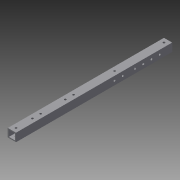
# Autodesk Inventor part: mounting block
Saved by Autodesk Inventor 2015 SP1 (Build 190203100, 203)
## iProperties
Created: 2015-01-16
Part Number: mounting block
Material: Generic
Document SubType Name: Modeling
Designer: Jarod
Density: 1 g/cm^3
Appearance: Default
Author: Jarod
Autodesk Inventor part; units mm, degrees
ref_plane "YZ Plane" through (0, 0, 0) normal (1, 0, 0) x (0, 1, 0)
ref_plane "XZ Plane" through (0, 0, 0) normal (0, 1, 0) x (-1, 0, 0)
ref_plane "XY Plane" through (0, 0, 0) normal (0, 0, 1) x (1, 0, 0)
sketch "Sketch1" plane through (0, 0, 0) normal (0, 0, 1) x (1, 0, 0)
  line L0 (0, 0) -> (25.4, 0)
  line L1 (25.4, 0) -> (25.4, 25.4)
  line L2 (25.4, 25.4) -> (0, 25.4)
  line L3 (0, 25.4) -> (0, 0)
  line L4 (3.175, 3.175) -> (22.225, 3.175)
  line L5 (22.225, 3.175) -> (22.225, 22.225)
  line L6 (22.225, 22.225) -> (3.175, 22.225)
  line L7 (3.175, 22.225) -> (3.175, 3.175)
  dimension "d0" = 25.4
  dimension "d1" = 25.4
  dimension "d2" = 19.05
  dimension "d3" = 19.05
  dimension "d4" = 3.175
  dimension "d5" = 3.175
  constraints: 16 end point, 4 parallel, 2 horizontal, 2 perpendicular
  measures "d0" distance of L2.end L1.end
  measures "d1" distance of L1.end L0.end
  measures "d2" distance of L6.end L5.end
  measures "d3" distance of L5.end L4.end
  measures "d4" distance between parallel lines of L0 L4
  measures "d5" distance between parallel lines of L3 L7
extrude "Extrusion1" add sketch "Sketch1" along normal blind 304.8
sketch "Sketch2" plane through (0, 25.4, 0) normal (0, 1, 0) x (1, 0, 0)
  line L0 (25.4, 0) -> (0, 0) projected
  line L1 (0, 0) -> (0, -304.8) projected
  line L2 (25.4, -304.8) -> (0, -304.8) projected
  line L3 (25.4, 0) -> (25.4, -304.8) projected
  point P0 (12.7, -292.1)
  point P1 (12.7, -12.7)
  point P2 (12.7, -165.1)
  dimension "d8" = 12.7
  dimension "d9" = 12.7
  dimension "d10" = 12.7
  dimension "d11" = 12.7
  dimension "d32" = 12.7
  dimension "d33" = 139.7
  measures "d8" distance from line of L1 point (12.7, -12.7)
  measures "d9" distance from line of L0 point (12.7, -12.7)
  measures "d10" distance from line of L2 point (12.7, -292.1)
  measures "d11" distance from line of point (12.7, -292.1) L1
  measures "d32" distance from line of L1 point (12.7, -165.1)
  measures "d33" distance from line of L2 point (12.7, -165.1)
sketch "Sketch3" plane through (25.4, 0, 0) normal (1, 0, 0) x (0, 0, -1)
  line L0 (0, 0) -> (-304.8, 0) projected
  line L1 (0, 0) -> (0, 25.4) projected
  point P0 (-38.1, 12.7)
  point P1 (-63.5, 12.7)
  point P2 (-88.9, 12.7)
  dimension "d19" = 12.7
  dimension "d20" = 12.7
  dimension "d21" = 12.7
  dimension "d22" = 38.1
  dimension "d23" = 88.9
  dimension "d24" = 63.5
  measures "d19" distance from line of L0 point (-38.1, 12.7)
  measures "d20" distance from line of L0 point (-63.5, 12.7)
  measures "d21" distance from line of L0 point (-88.9, 12.7)
  measures "d22" distance from line of L1 point (-38.1, 12.7)
  measures "d23" distance from line of L1 point (-88.9, 12.7)
  measures "d24" distance from line of L1 point (-63.5, 12.7)
hole "Hole2" at (25.4, 12.7, 38.1) at (25.4, 12.7, 63.5) at (25.4, 12.7, 88.9) direction (-1, 0, 0) diameter 6.35 end through all
hole "Hole3" at (12.7, 25.4, 292.1) at (12.7, 25.4, 12.7) at (12.7, 25.4, 165.1) direction (0, -1, 0) diameter 6.35 end through all
sketch "Sketch4" plane through (25.4, 0, 0) normal (1, 0, 0) x (0, 0, -1)
  circle A0 centre (-63.5, 12.7) radius 3.175 projected
  circle A1 centre (-38.1, 12.7) radius 3.175 projected
  circle A2 centre (-88.9, 12.7) radius 3.175 projected
  line L0 (0, 0) -> (0, 25.4) projected
  line L1 (0, 25.4) -> (-304.8, 25.4) projected
  line L2 (-304.8, 0) -> (-304.8, 25.4) projected
  line L3 (0, 0) -> (-304.8, 0) projected
  point P0 (-177.8, 12.7)
  point P1 (-114.3, 12.7)
  point P2 (-152.4, 12.7)
  dimension "d41" = 127
  dimension "d42" = 190.5
  dimension "d43" = 152.4
  dimension "d44" = 12.7
  dimension "d45" = 12.7
  dimension "d46" = 12.7
  measures "d41" distance from line of point (-177.8, 12.7) L2
  measures "d42" distance from line of point (-114.3, 12.7) L2
  measures "d43" distance from line of L2 point (-152.4, 12.7)
  measures "d44" distance from line of L3 point (-177.8, 12.7)
  measures "d45" distance from line of L3 point (-152.4, 12.7)
  measures "d46" distance from line of L3 point (-114.3, 12.7)
hole "Hole4" at (25.4, 12.7, 177.8) at (25.4, 12.7, 114.3) at (25.4, 12.7, 152.4) direction (-1, 0, 0) diameter 6.35 end through all
sketch "Sketch5" plane through (0, 0, 304.8) normal (0, 0, 1) x (1, 0, 0)
  line L0 (3.175, 3.175) -> (3.175, 22.225) projected
  line L1 (3.175, 22.225) -> (22.225, 22.225) projected
  line L2 (22.225, 22.225) -> (22.225, 3.175) projected
  line L3 (22.225, 3.175) -> (3.175, 3.175) projected
  line L4 (0, 0) -> (25.4, 0) projected
  line L5 (25.4, 0) -> (25.4, 25.4) projected
  line L6 (25.4, 25.4) -> (0, 25.4) projected
  line L7 (0, 25.4) -> (0, 0) projected
extrude "Extrusion2" add sketch "Sketch5" along normal blind 177.8
sketch "Sketch6" plane through (0, 25.4, 0) normal (0, 1, 0) x (1, 0, 0)
  line L0 (25.4, -482.6) -> (0, -482.6) projected
  line L1 (25.4, 0) -> (25.4, -482.6) projected
  point P0 (12.7, -469.9)
  point P1 (12.7, -419.1)
  dimension "d56" = 12.7
  dimension "d57" = 12.7
  dimension "d65" = 63.5
  dimension "d66" = 12.7
  measures "d56" distance from line of point (12.7, -469.9) L0
  measures "d57" distance from line of L1 point (12.7, -469.9)
  measures "d65" distance from line of L0 point (12.7, -419.1)
  measures "d66" distance from line of L1 point (12.7, -419.1)
hole "Hole6" at (12.7, 25.4, 469.9) at (12.7, 25.4, 419.1) direction (0, -1, 0) diameter 6.35 depth 25.4 tip angle 118
sketch "Sketch7" plane through (0, 25.4, 0) normal (0, 1, 0) x (1, 0, 0)
  circle A0 centre (12.7, -469.9) radius 3.175 projected
  circle A1 centre (12.7, -419.1) radius 3.175 projected
  circle A2 centre (12.7, -12.7) radius 3.175 projected
  circle A3 centre (12.7, -292.1) radius 3.175 projected
  circle A4 centre (12.7, -165.1) radius 3.175 projected
  line L0 (25.4, 0) -> (0, 0) projected
  line L1 (0, 0) -> (0, -482.6) projected
  line L2 (25.4, -482.6) -> (0, -482.6) projected
  line L3 (25.4, 0) -> (25.4, -482.6) projected
  point P0 (12.7, -393.7)
  point P1 (12.7, -317.5)
  dimension "d74" = 12.7
  dimension "d75" = 12.7
  dimension "d76" = 88.9
  dimension "d77" = 165.1
  measures "d74" distance from line of L3 point (12.7, -393.7)
  measures "d75" distance from line of L3 point (12.7, -317.5)
  measures "d76" distance from line of L2 point (12.7, -393.7)
  measures "d77" distance from line of point (12.7, -317.5) L2
hole "Hole7" at (12.7, 25.4, 393.7) at (12.7, 25.4, 317.5) direction (0, -1, 0) diameter 6.35 end through all
body "Solid1"
